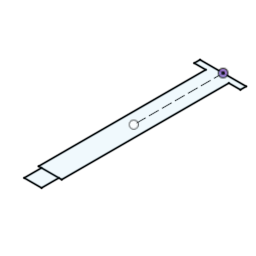
BLDC Mount (Autodesk Fusion 360 design; units mm, degrees)
Autodesk Fusion 360 part; units mm, degrees
sketch "스케치1" plane through (0, 0, 0) normal (0, 0, 1) x (1, 0, 0)
  line L0 (0, 0) -> (109, 0)
  line L1 (109, 0) -> (109, 80)
  line L2 (109, 80) -> (0, 80)
  line L3 (0, 80) -> (0, 0)
  line L4 (0, 40) -> (109, 40) construction
  line L5 (2, 47.8266) -> (6, 47.8266)
  line L6 (6, 47.8266) -> (6, 32.1734)
  line L7 (6, 32.1734) -> (2, 32.1734)
  line L8 (2, 32.1734) -> (2, 47.8266)
  line L9 (66, 64.6) -> (101, 64.6)
  line L10 (101, 64.6) -> (101, 15.4)
  line L11 (101, 15.4) -> (66, 15.4)
  line L12 (66, 15.4) -> (66, 64.6)
  circle A0 centre (3, 8) radius 1.5
  circle A1 centre (3, 72) radius 1.5
  line L13 (73.5, 72.3) -> (93.5, 72.3) construction
  line L14 (83.5, 72.3) -> (83.5, 64.6) construction
  circle A2 centre (73.5, 72.3) radius 1.5
  circle A3 centre (93.5, 72.3) radius 1.5
  circle A4 centre (73.5, 7.7) radius 1.5
  circle A5 centre (93.5, 7.7) radius 1.5
  dimension "d1" = 80
  dimension "d2" = 49.2
  dimension "d3" = 35
  dimension "d4" = 2
  dimension "d11" = 4
  dimension "d12" = 60
  dimension "d13" = 8
  dimension "d49" = 3
  dimension "d50" = 8
  dimension "d51" = 3
  dimension "d52" = 20
  dimension "d53" = 3
  constraint horizontal L0
  constraint vertical L1
  constraint horizontal L2
  constraint vertical L3
  constraint coincident L0.start L3.end
  constraint midpoint L3 L4.start
  constraint midpoint L1 L4.end
  constraint horizontal L5
  constraint vertical L6
  constraint horizontal L7
  constraint vertical L8
  constraint symmetric L4 L5 L7
  constraint horizontal L9
  constraint vertical L10
  constraint horizontal L11
  constraint vertical L12
  constraint symmetric L4 L9 L11
  constraint equal A0 A1
  constraint symmetric L4 A0 A1
  constraint horizontal L13
  constraint midpoint L13 L14.start
  constraint midpoint L9 L14.end
  constraint vertical L14
  constraint coincident L13.start A2.centre
  constraint coincident L13.end A3.centre
  constraint equal A2 A3
  constraint equal A4 A5
  constraint equal A2 A5
  constraint symmetric L4 A2 A4
  constraint symmetric L4 A3 A5
  measures "d1" distance of L0.start L2.end
  measures "d2" distance of L9.end L10.end
  measures "d3" distance of L9.start L9.end
  measures "d4" distance of L3 L8
  measures "d11" distance of L5.start L5.end
  measures "d12" distance of L6 L12
  measures "d13" distance of L1 L10
  measures "d49" diameter of A0
  measures "d50" distance of L0 A0.centre
  measures "d51" distance of L3 A0.centre
  measures "d52" distance of L13.start L13.end
  measures "d53" diameter of A2
sketch "스케치2" plane through (0, 0, 0) normal (1, 0, 0) x (0, 1, 0)
  line L0 (0, 0) -> (80, 0)
  line L1 (80, 0) -> (80, 8)
  line L2 (40, 0) -> (40, 28.6) construction
  circle A0 centre (40, 28.6) radius 24.6 construction
  circle A1 centre (40, 28.6) radius 25.1
  circle A2 centre (40, 28.6) radius 33.1 construction
  line L3 (0, 0) -> (0, 8)
  line L4 (6.9, 8) -> (6.9, 28.6)
  line L5 (73.1, 8) -> (73.1, 28.6)
  arc A3 (73.1, 28.6) -> (6.9, 28.6) centre (40, 28.6) ccw
  line L6 (6.9, 8) -> (0, 8)
  line L7 (73.1, 8) -> (80, 8)
  dimension "d15" = 28.6
  dimension "d16" = 49.2
  dimension "d17" = 0.5
  dimension "d21" = 8
  dimension "d22" = 80
  dimension "d44" = 8
  constraint coincident L0.start L3.start
  constraint horizontal L0
  constraint perpendicular L0 L1
  constraint midpoint L0 L2.start
  constraint perpendicular L0 L2
  constraint coincident L2.end A0.centre
  constraint concentric A0 A1
  constraint concentric A1 A2
  constraint perpendicular L0 L3
  constraint coincident A2 L4.end
  constraint coincident A2 L5.end
  constraint tangent A2 L5
  constraint tangent A2 L4
  constraint equal L1 L3
  constraint tangent L4 A3
  constraint tangent L5 A3
  constraint horizontal L6
  constraint vertical L4
  constraint horizontal L7
  constraint vertical L5
  measures "d15" distance of L2.start L2.end
  measures "d16" diameter of A0
  measures "d17" distance of A0 A1
  measures "d21" distance of A1 A2
  measures "d22" distance of L0.start L0.end
  measures "d44" distance of L0.end L1.end
sketch "스케치3" plane through (0, 0, 0) normal (1, 0, 0) x (0, 1, 0)
  line L0 (0, 0) -> (80, 0)
  line L1 (80, 0) -> (80, 8)
  line L2 (40, 0) -> (40, 28.6) construction
  circle A0 centre (40, 28.6) radius 12.5 construction
  line L3 (52.5, 28.6) -> (27.5, 28.6) construction
  line L4 (40, 28.6) -> (40, 41.1) construction
  circle A1 centre (40, 41.1) radius 1.5
  circle A2 centre (27.5, 28.6) radius 1.5
  circle A3 centre (52.5, 28.6) radius 1.5
  circle A4 centre (40, 16.1) radius 1.5
  circle A5 centre (40, 28.6) radius 20.5 construction
  line L5 (80, 8) -> (56.6589, 40.547)
  line L6 (0, 0) -> (0, 8)
  line L7 (0, 8) -> (23.3411, 40.547)
  arc A6 (56.6589, 40.547) -> (23.3411, 40.547) centre (40, 28.6) ccw
  line L8 (58.9035, 23.6898) -> (70.1554, 8)
  line L9 (70.1554, 8) -> (43.2137, 8)
  line L10 (43.2137, 8) -> (58.9035, 23.6898)
  line L11 (36.7863, 8) -> (9.8446, 8)
  line L12 (9.8446, 8) -> (21.0965, 23.6898)
  line L13 (21.0965, 23.6898) -> (36.7863, 8)
  line L14 (80, 0) -> (0, 0)
  circle A7 centre (40, 28.6) radius 4.5
  dimension "d23" = 80
  dimension "d24" = 28.6
  dimension "d25" = 25
  dimension "d26" = 3
  dimension "d27" = 8
  dimension "d28" = 8
  dimension "d29" = 8
  dimension "d30" = 8
  dimension "d31" = 45
  dimension "d32" = 8
  dimension "d33" = 8
  constraint coincident L0.start L6.start
  constraint horizontal L0
  constraint perpendicular L0 L1
  constraint midpoint L0 L2.start
  constraint perpendicular L0 L2
  constraint coincident L2.end A0.centre
  constraint coincident A0 L3.start
  constraint coincident A0 L3.end
  constraint perpendicular L2 L3
  constraint coincident A0 L4.end
  constraint perpendicular L3 L4
  constraint coincident L4.end A1.centre
  constraint coincident L3.end A2.centre
  constraint coincident L3.start A3.centre
  constraint coincident A0 A4.centre
  constraint coincident L2 A4.centre
  constraint equal A1 A2
  constraint equal A1 A4
  constraint equal A1 A3
  constraint concentric A0 A5
  constraint coincident A5 L5.end
  constraint perpendicular L0 L6
  constraint coincident A5 L7.end
  constraint tangent A5 L5
  constraint symmetric L2 L5 L7
  constraint tangent L7 A6
  constraint perpendicular L1 L9
  constraint parallel L9 L11
  constraint parallel L7 L12
  constraint parallel L5 L8
  constraint collinear L9 L11
  constraint symmetric L2 L8 L12
  constraint symmetric L2 L10 L13
  constraint concentric A0 A7
  measures "d23" distance of L0.start L0.end
  measures "d24" distance of L2.start L2.end
  measures "d25" diameter of A0
  measures "d26" diameter of A1
  measures "d27" distance of L0.end L1.end
  measures "d28" distance of A0 A5
  measures "d29" distance of L5 L8
  measures "d30" distance of L9 L14
  measures "d31" angle of L9 L10
  measures "d32" distance of L3.start L10
  measures "d33" distance of A0 A7
sketch "스케치4" plane through (0, 0, 0) normal (1, 0, 0) x (0, 1, 0)
  line L0 (0, 0) -> (80, 0)
  line L1 (80, 0) -> (80, 8)
  line L2 (40, 0) -> (40, 28.6) construction
  circle A0 centre (40, 28.6) radius 3.5
  circle A1 centre (40, 28.6) radius 6
  circle A2 centre (40, 28.6) radius 14 construction
  line L3 (0, 0) -> (0, 8)
  line L4 (0, 8) -> (26, 8)
  line L5 (26, 8) -> (26, 28.6)
  line L6 (80, 8) -> (54, 8)
  line L7 (54, 8) -> (54, 28.6)
  arc A3 (54, 28.6) -> (26, 28.6) centre (40, 28.6) ccw
  line L8 (54, 8) -> (26, 8)
  dimension "d34" = 80
  dimension "d35" = 8
  dimension "d36" = 28.6
  dimension "d37" = 7
  dimension "d38" = 12
  dimension "d39" = 8
  constraint coincident L0.start L3.start
  constraint horizontal L0
  constraint perpendicular L0 L1
  constraint midpoint L0 L2.start
  constraint perpendicular L0 L2
  constraint coincident L2.end A0.centre
  constraint concentric A0 A2
  constraint perpendicular L0 L3
  constraint equal L1 L3
  constraint perpendicular L3 L4
  constraint coincident A2 L5.end
  constraint tangent A2 L5
  constraint perpendicular L1 L6
  constraint coincident A2 L7.end
  constraint tangent A2 L7
  constraint vertical L7
  constraint vertical L5
  constraint tangent L7 A3
  measures "d34" distance of L0.start L0.end
  measures "d35" distance of L0.end L1.end
  measures "d36" distance of L2.start L2.end
  measures "d37" diameter of A0
  measures "d38" diameter of A1
  measures "d39" distance of A1 A2
extrude "돌출1" add sketch "스케치2" along normal blind 35 makes body 1
move_body "정렬1" bodies 1 to x (1, 0, 0) y (0, 1, 0) z (0, 0, 1) at (66, 0, 0)
extrude "돌출2" add sketch "스케치3" along normal blind 8 separate body makes body 2
move_body "정렬2" bodies 2 to x (1, 0, 0) y (0, 1, 0) z (0, 0, 1) at (101, 0, 0)
combine "결합1" operation add target body 1 tool bodies 2
extrude "돌출3" add sketch "스케치4" along normal blind 2 separate body contours L0 L1 L3 L4 L6 L8 | L5 L7 A3 L8 | A1 makes body 3
extrude "돌출4" add sketch "스케치4" along normal blind 6 separate body contours L0 L1 L3 L4 L6 L8 | L5 L7 A3 L8 makes body 4
combine "결합3" operation add target body 4 tool bodies 3
extrude "돌출5" add sketch "스케치1" along normal blind 8 separate body contours A0 | A1 | A2 | A3 | A4 | A5 makes body 5 at (94.9981, 7.6252, 5.3333) makes body 6 at (4.3822, 72.5827, 5.3333) makes body 7 at (74.8822, 72.8827, 5.3333) makes body 8 at (74.9981, 7.6252, 5.3333) makes body 9 at (4.4981, 7.9252, 5.3333) makes body 10 at (94.8822, 72.8827, 5.3333)
combine "결합4" operation cut target body 1 tool bodies 8
combine "결합5" operation cut target body 1 tool bodies 7
combine "결합6" operation cut target body 1 tool bodies 10
combine "결합7" operation cut target body 1 tool bodies 5
combine "결합8" operation cut target body 4 tool bodies 9
combine "결합9" operation cut target body 4 tool bodies 6
sketch "스케치5" plane through (0, 0, 0) normal (0, 1, 0) x (1, 0, 0)
  circle A0 centre (0, 0) radius 6 construction
  line L0 (-4.2426, -4.2426) -> (4.2426, -4.2426) construction
  line L1 (4.2426, -4.2426) -> (4.2426, 4.2426) construction
  line L2 (4.2426, 4.2426) -> (-4.2426, 4.2426) construction
  line L3 (-4.2426, 4.2426) -> (-4.2426, -4.2426) construction
  circle A1 centre (-4.2426, -4.2426) radius 1.5
  circle A2 centre (4.2426, -4.2426) radius 1.5
  circle A3 centre (4.2426, 4.2426) radius 1.5
  circle A4 centre (-4.2426, 4.2426) radius 1.5
  circle A5 centre (0, 0) radius 7.5 construction
  circle A6 centre (0, 0) radius 9.5
  dimension "d56" = 12
  dimension "d57" = 3
  dimension "d58" = 2
  constraint coincident A0.centre A5.centre
  constraint coincident A0 L0.start
  constraint coincident A0 L0.end
  constraint horizontal L0
  constraint coincident A0 L1.end
  constraint perpendicular L0 L1
  constraint perpendicular L1 L2
  constraint vertical L3
  constraint equal L0 L1
  constraint coincident L0.start L3.end
  constraint coincident L0.end L1.start
  constraint coincident L1.end L2.start
  constraint coincident L2.end L3.start
  constraint equal A1 A4
  constraint equal A1 A2
  constraint equal A1 A3
  constraint concentric A0 A5
  constraint tangent A2 A5
  constraint concentric A0 A6
  measures "d56" diameter of A0
  measures "d57" diameter of A1
  measures "d58" distance of A5 A6
sketch "스케치6" plane through (0, 0, 0) normal (0, 0, 1) x (1, 0, 0)
  line L0 (0, 0) -> (0, -31) construction
  line L1 (0, 0) -> (8, 0)
  line L2 (8, 0) -> (8, -2)
  line L3 (8, -2) -> (4, -2)
  line L4 (0, 0) -> (-8, 0)
  line L5 (-8, 0) -> (-8, -2)
  line L6 (-8, -2) -> (-4, -2)
  line L7 (4, -2) -> (4, -60)
  line L8 (4, -60) -> (-4, -60)
  line L9 (-4, -60) -> (-4, -2)
  line L10 (3, -60) -> (3, -66)
  line L11 (3, -66) -> (-3, -66)
  line L12 (-3, -66) -> (-3, -60)
  dimension "d59" = 8
  dimension "d60" = 2
  dimension "d61" = 6
  dimension "d62" = 8
  dimension "d63" = 60
  dimension "d64" = 6
  constraint coincident L0.start L1.start
  constraint vertical L0
  constraint perpendicular L0 L1
  constraint perpendicular L1 L2
  constraint perpendicular L2 L3
  constraint perpendicular L0 L4
  constraint perpendicular L4 L5
  constraint perpendicular L0 L6
  constraint equal L1 L4
  constraint equal L2 L5
  constraint perpendicular L3 L7
  constraint perpendicular L7 L8
  constraint perpendicular L6 L9
  constraint symmetric L0 L7 L9
  constraint coincident L8 L10.start
  constraint perpendicular L8 L10
  constraint perpendicular L0 L11
  constraint coincident L8 L12.end
  constraint symmetric L0 L10 L12
  measures "d59" distance of L0.start L1.end
  measures "d60" distance of L1.end L2.end
  measures "d61" distance of L10.end L11.end
  measures "d62" distance of L7 L9
  measures "d63" distance of L1 L8
  measures "d64" distance of L11.end L12.end
hidden bodies 1 4
equation "d4 = thn"
equation "thn = 2 mm"
equation "thk = 8 mm"
equation "bearing_d = 6 mm"
equation "bearing_D = 12 mm"
equation "bearing_h = 4 mm"
equation "dcc_rate = 20"
equation "d11 = bearing_h"
equation "d13 = thk"
equation "d15 = moter_rad / 2 + thk / 2"
equation "d17 = error"
equation "error = 0.5 mm"
equation "moter_rad = 49.2 mm"
equation "d21 = thk"
equation "d22 = d1"
equation "d23 = d1"
equation "d24 = d15"
equation "d27 = thk"
equation "d28 = thk"
equation "d29 = thk"
equation "d30 = thk"
equation "d32 = thk"
equation "d33 = thk"
equation "d34 = d1"
equation "d35 = thk"
equation "d36 = d15"
equation "d37 = bearing_d + error * 2"
equation "d38 = bearing_D"
equation "d39 = thk"
equation "d42 = thk"
equation "d44 = thk"
equation "d45 = thn"
equation "d47 = thn + bearing_h"
equation "d50 = thk"
equation "d51 = ( thn + bearing_h ) / 2"
equation "d54 = thk"
equation "d58 = thn"
equation "d59 = ( 12 / 2 ) * 1 mm + thn"
equation "d60 = thn"
equation "d61 = bearing_d"
equation "d63 = d12"
equation "d64 = thn + bearing_h"
